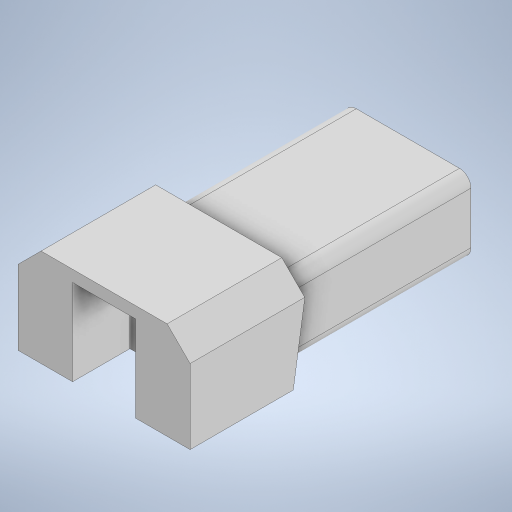
# Autodesk Inventor part: gunv1
Saved by Autodesk Inventor 2024 (Build 280153000, 153)
## iProperties
Created: 2025-05-22
Part Number: gunv1
Material: Ogólny
Document SubType Name: Modeling
Designer: Victoria
Density: 1 g/cm^3
Appearance: Domyślna
Author: Victoria
Autodesk Inventor part; units mm, degrees
ref_plane "YZ Plane" through (0, 0, 0) normal (1, 0, 0) x (0, 1, 0)
ref_plane "XZ Plane" through (0, 0, 0) normal (0, 1, 0) x (-1, 0, 0)
ref_plane "XY Plane" through (0, 0, 0) normal (0, 0, 1) x (1, 0, 0)
sketch "Szkic1" plane through (0, 0, 0) normal (0, 0, 1) x (1, 0, 0)
  line L0 (-15, -8.5) -> (15, -8.5)
  line L1 (15, -8.5) -> (15, 4.5)
  line L2 (11, 8.5) -> (-11, 8.5)
  line L3 (-15, 4.5) -> (-15, -8.5)
  line L4 (-15, -8.5) -> (15, 8.5) construction
  line L5 (15, -8.5) -> (-15, 8.5) construction
  line L6 (-13, 6.5) -> (13, 6.5)
  line L7 (13, 6.5) -> (13, -6.5)
  line L8 (13, -6.5) -> (-13, -6.5)
  line L9 (-13, -6.5) -> (-13, 6.5)
  line L10 (-5.5, -6.5) -> (5.5, -6.5)
  line L11 (5.5, -6.5) -> (5.5, 6.5)
  line L12 (5.5, 6.5) -> (-5.5, 6.5)
  line L13 (-5.5, 6.5) -> (-5.5, -6.5)
  line L14 (-5.5, -6.5) -> (5.5, 6.5) construction
  line L15 (5.5, -6.5) -> (-5.5, 6.5) construction
  line L16 (-5.5, -6.5) -> (-5.5, -8.5)
  line L17 (5.5, -6.5) -> (5.5, -8.5)
  line L18 (-11, 8.5) -> (-15, 4.5)
  line L19 (11, 8.5) -> (15, 4.5)
  point P0 (0, 0)
  dimension "d0" = 30
  dimension "d1" = 17
  dimension "d2" = 2
  dimension "d3" = 11
  dimension "d4" = 4
  dimension "d5" = 4
  dimension "d6" = 4
  dimension "d7" = 4
  constraints: 40 end point, 8 point on line, 6 parallel, 4 midpoint, 4 perpendicular, 2 horizontal, 3 other
  measures "d0" distance of L5.end L4.end
  measures "d1" distance of L4.end L0.end
  measures "d2" distance between parallel lines of L2 L6
  measures "d3" distance of L12.end L11.end
  measures "d4" distance of L2.end L5.end
  measures "d5" distance of L3.start L5.end
  measures "d6" distance of L2.start L4.end
  measures "d7" distance of L1.end L4.end
extrude "Wyciągnięcie proste1" add sketch "Szkic1" along normal blind 10 contours L3 L18 L9 L8 L16 L0 | L17 L8 L7 L19 L1 L0 | L8 L9 L6 L13 | L18 L2 L19 L6 | L11 L6 L7 L8
sketch "Szkic2" plane through (0, 0, 0) normal (0, 0, -1) x (-1, 0, 0)
  line L0 (5.5, 6.5) -> (-5.5, 6.5) projected
  line L1 (5.5, -8.5) -> (5.5, 6.5) projected
  line L2 (15, -8.5) -> (5.5, -8.5) projected
  line L3 (15, 4.5) -> (15, -8.5) projected
  line L4 (11, 8.5) -> (15, 4.5) projected
  line L5 (-11, 8.5) -> (11, 8.5) projected
  line L6 (-15, 4.5) -> (-11, 8.5) projected
  line L7 (-15, -8.5) -> (-15, 4.5) projected
  line L8 (-5.5, -8.5) -> (-15, -8.5) projected
  line L9 (-5.5, 6.5) -> (-5.5, -8.5) projected
  line L10 (-5.5, -8.5) -> (5.5, -8.5)
  point P0 (0, 0)
  constraints: 2 end point, 1 horizontal
extrude "Wyciągnięcie proste2" add sketch "Szkic2" along normal blind 10
sketch "Szkic3" plane through (0, 0, -10) normal (0, 0, -1) x (-1, 0, 0)
  line L0 (15, -8.5) -> (15, 4.5) projected
  line L1 (15, 4.5) -> (11, 8.5) projected
  line L2 (11, 8.5) -> (-11, 8.5) projected
  line L3 (-11, 8.5) -> (-15, 4.5) projected
  line L4 (-15, 4.5) -> (-15, -8.5) projected
  line L5 (-15, -8.5) -> (15, -8.5) projected
  line L6 (10.1716, 6.5) -> (13, 3.6716)
  line L7 (13, 3.6716) -> (13, -6.5)
  line L8 (13, -6.5) -> (-13, -6.5)
  line L9 (-13, -6.5) -> (-13, 3.6716)
  line L10 (-13, 3.6716) -> (-10.1716, 6.5)
  line L11 (-10.1716, 6.5) -> (10.1716, 6.5)
  line L12 (-13, -6.5) -> (-13, -8.5)
  line L13 (13, -6.5) -> (13, -8.5)
  point P0 (0, 0)
  dimension "d12" = 2
  constraints: 16 end point, 2 perpendicular, 2 point on line, 5 other
  measures "d12" distance between parallel lines of L1 L6
extrude "Wyciągnięcie proste3" cut sketch "Szkic3" against normal blind 7 contours L5 L12 L8 L13 | L8 L9 L10 L11 L6 L7
sketch "Szkic4" plane through (15, -8.5, 10) normal (1, 0, 0) x (0, 0, -1)
  line L0 (20, 0) -> (0, 0) projected
  line L1 (20, 0) -> (18, 0)
  line L2 (18, 0) -> (20, 12.8915)
  line L3 (20, 12.8915) -> (20, 0)
  point P0 (10, 8.5)
  dimension "d15" = 2
  constraints: 6 end point, 1 perpendicular, 1 point on line
  measures "d15" distance of L0.start L1.end
extrude "Wyciągnięcie proste4" cut sketch "Szkic4" against normal through all
sketch "Szkic6" plane through (0, 0, -3) normal (0, 0, -1) x (-1, 0, 0)
  line L0 (-11, 4.5) -> (11, 4.5)
  line L1 (11, 4.5) -> (11, -17.5)
  line L2 (11, -17.5) -> (-11, -17.5)
  line L3 (-11, -17.5) -> (-11, 4.5)
  line L4 (13, -8.5) -> (-13, -8.5) projected
  line L5 (-11, 4.5) -> (11, 4.5)
  line L6 (11, 4.5) -> (11, -8.5)
  line L7 (11, -8.5) -> (-11, -8.5)
  line L8 (-11, -8.5) -> (-11, 4.5)
  point P0 (0, 0)
  dimension "d18" = 22
  dimension "d19" = 22
  constraints: 16 end point, 4 parallel, 2 horizontal, 2 perpendicular, 2 point on line
  measures "d18" distance of L1.end L2.end
  measures "d19" distance of L0.end L1.end
extrude "Wyciągnięcie proste5" add sketch "Szkic6" along normal blind 40 contours L0 L1 L4 L3
fillet "Zaokrąglenie1" radius 2 4 edges at (11, 4.5, -23) (11, -8.5, -23) (-11, -8.5, -23) (-11, 4.5, -23)
sketch "Szkic7" plane through (0, 0, -43) normal (0, 0, -1) x (-1, 0, 0)
  line L0 (11, -6.5) -> (11, 2.5) projected
  arc A0 (11, 2.5) -> (9, 4.5) centre (9, 2.5) ccw projected
  line L1 (9, 4.5) -> (-9, 4.5) projected
  arc A1 (-9, 4.5) -> (-11, 2.5) centre (-9, 2.5) ccw projected
  line L2 (-11, 2.5) -> (-11, -6.5) projected
  arc A2 (-11, -6.5) -> (-9, -8.5) centre (-9, -6.5) ccw projected
  line L3 (-9, -8.5) -> (9, -8.5) projected
  arc A3 (9, -8.5) -> (11, -6.5) centre (9, -6.5) ccw projected
  line L4 (11, -6.5) -> (11, 2.5) projected
  line L5 (-7, 2.5) -> (7, 2.5)
  line L6 (9, 0.5) -> (9, -4.5)
  line L7 (7, -6.5) -> (-7, -6.5)
  line L8 (-9, -4.5) -> (-9, 0.5)
  arc A4 (-7, 2.5) -> (-9, 0.5) centre (-7, 0.5) ccw
  arc A5 (-9, -4.5) -> (-7, -6.5) centre (-7, -4.5) ccw
  arc A6 (7, -6.5) -> (9, -4.5) centre (7, -4.5) ccw
  arc A7 (9, 0.5) -> (7, 2.5) centre (7, 0.5) ccw
  point P0 (0, 0)
  dimension "d23" = 2
  dimension "d24" = 2
  constraints: 8 end point, 8 point on circle, 8 tangent, 4 centre point, 3 equal radius, 3 other
  measures "d23" distance between parallel lines of L1 L5
  measures "d24" radius of A4
extrude "Wyciągnięcie proste6" cut sketch "Szkic7" against normal blind 25 contours L5 A7 L6 A6 L7 A5 L8 A4
equation "\"d5\" = d4"
equation "\"d6\" = d4"
equation "\"d7\" = d6"
